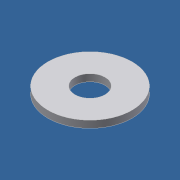
# Autodesk Inventor part: BN1075_M4
Saved by Autodesk Inventor 2021.2 (Build 252289000, 289)
## iProperties
Created: 2021-02-22
Part Number: BN1075_M4
Project: Nom Projet
Material: PA6 (Polyamide 6)
Description: Rondelle en polyamide
Document SubType Name: Modeling
Designer: Jean-Marc.VULLIAMY
Density: 1.13 g/cm^3
Appearance: Par défaut
Mass: 0.11139 g
Surface Area: 2.48359 cm^2
Volume: 0.0985753 cm^3
Authority: B&R 864369
Material number: ---
Author: Jean-Marc.VULLIAMY
Autodesk Inventor part; units mm, degrees
ref_plane "Plan YZ" through (0, 0, 0) normal (1, 0, 0) x (0, 1, 0)
ref_plane "Plan XZ" through (0, 0, 0) normal (0, 1, 0) x (-1, 0, 0)
ref_plane "Plan XY" through (0, 0, 0) normal (0, 0, 1) x (1, 0, 0)
sketch "Esquisse1" plane through (0, 0, 0) normal (0, 0, 1) x (1, 0, 0)
  circle A0 centre (0, 0) radius 2.15
  circle A1 centre (0, 0) radius 6
  dimension "d0" = 12
  dimension "d1" = 4.3
  constraints: 2 centre point, 2 coincident
  measures "d0" diameter of A1
  measures "d1" diameter of A0
extrude "Extrusion1" add sketch "Esquisse1" along normal blind 1
